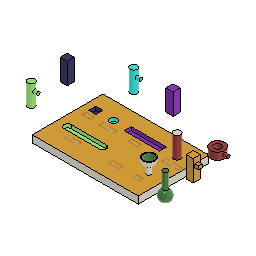
assembly_joint_practical (Autodesk Fusion 360 design; units mm, degrees)
part number: Joing-plate
part number: Rigid part
part number: Revolute part
part number: Slider part
part number: Cylindrical
part number: Pin-Slot part
part number: Planar part
part number: Ball part
Autodesk Fusion 360 part; units mm, degrees
sketch "スケッチ1" plane through (0, 0, 0) normal (0, 1, 0) x (1, 0, 0) in component "Joint-plate"
  line L0 (75, -50) -> (-75, -50)
  line L1 (-75, -50) -> (-75, 50)
  line L2 (-75, 50) -> (75, 50)
  line L3 (75, 50) -> (75, -50)
  line L4 (75, -50) -> (-75, 50) construction
  line L5 (-75, -50) -> (75, 50) construction
  dimension "d1" = 100
  dimension "d2" = 150
  constraint perpendicular L0 L1
  constraint parallel L0 L2
  constraint parallel L1 L3
  constraint horizontal L0
  constraint coincident L4 origin
  constraint coincident L5 origin
  measures "d1" distance of L0.end L1.end
  measures "d2" distance of L1.end L2.end
extrude "押し出し1" add sketch "スケッチ1" along normal blind 10 makes body 1 in component "Joint-plate"
sketch "スケッチ2" plane through (0, 10, 0) normal (0, 1, 0) x (-1, 0, 0) in component "Joint-plate"
  line L0 (-75, -50) -> (75, -50)
  line L1 (75, -50) -> (75, 50)
  line L2 (75, 50) -> (-75, 50)
  line L3 (-75, 50) -> (-75, -50)
  line L4 (65, -30) -> (55, -30)
  line L5 (55, -30) -> (55, -20)
  line L6 (55, -20) -> (65, -20)
  line L7 (65, -20) -> (65, -30)
  dimension "d5" = 10
  dimension "d6" = 20
  dimension "d7" = 10
  dimension "d8" = 10
  constraint horizontal L4
  constraint vertical L5
  constraint horizontal L6
  constraint vertical L7
  measures "d5" distance of L1 L7
  measures "d6" distance of L0 L4
  measures "d7" distance of L4.start L6.end
  measures "d8" distance of L5.end L6.end
extrude "押し出し2" cut sketch "スケッチ2" against normal blind 5 contours L4 L5 L6 L7 bodies 1 in component "Joint-plate"
sketch "スケッチ3" plane through (0, 10, 0) normal (0, 1, 0) x (-1, 0, 0) in component "Joint-plate"
  line L0 (55, -30) -> (55, -20)
  line L1 (55, -20) -> (65, -20)
  line L2 (65, -20) -> (65, -30)
  line L3 (65, -30) -> (55, -30)
  line L4 (-75, -50) -> (75, -50)
  line L5 (75, -50) -> (75, 50)
  line L6 (75, 50) -> (-75, 50)
  line L7 (-75, 50) -> (-75, -50)
  circle A0 centre (35, -25) radius 5
  dimension "d11" = 25
  dimension "d12" = 10
  dimension "d13" = 40
  measures "d11" distance of L4 A0.centre
  measures "d12" diameter of A0
  measures "d13" distance of L5 A0.centre
extrude "押し出し3" cut sketch "スケッチ3" against normal blind 5 contours A0 bodies 1 in component "Joint-plate"
sketch "スケッチ4" plane through (0, 10, 0) normal (0, 1, 0) x (-1, 0, 0) in component "Joint-plate"
  circle A0 centre (35, -25) radius 5
  line L0 (55, -30) -> (55, -20)
  line L1 (55, -20) -> (65, -20)
  line L2 (65, -20) -> (65, -30)
  line L3 (65, -30) -> (55, -30)
  line L4 (-75, -50) -> (75, -50)
  line L5 (75, -50) -> (75, 50)
  line L6 (75, 50) -> (-75, 50)
  line L7 (-75, 50) -> (-75, -50)
  line L8 (15, -30) -> (-35, -30)
  line L9 (-35, -30) -> (-35, -20)
  line L10 (-35, -20) -> (15, -20)
  line L11 (15, -20) -> (15, -30)
  dimension "d16" = 10
  dimension "d17" = 20
  dimension "d18" = 60
  dimension "d19" = 50
  constraint horizontal L8
  constraint vertical L9
  constraint horizontal L10
  constraint vertical L11
  measures "d16" distance of L8.start L10.end
  measures "d17" distance of L4 L8
  measures "d18" distance of L5 L11
  measures "d19" distance of L8.start L8.end
extrude "押し出し4" cut sketch "スケッチ4" against normal blind 5 contours L8 L9 L10 L11 bodies 1 in component "Joint-plate"
sketch "スケッチ5" plane through (0, 10, 0) normal (0, 1, 0) x (-1, 0, 0) in component "Joint-plate"
  line L0 (-35, -30) -> (-35, -20)
  line L1 (-35, -20) -> (15, -20)
  line L2 (15, -20) -> (15, -30)
  line L3 (15, -30) -> (-35, -30)
  circle A0 centre (35, -25) radius 5
  line L4 (55, -30) -> (55, -20)
  line L5 (55, -20) -> (65, -20)
  line L6 (65, -20) -> (65, -30)
  line L7 (65, -30) -> (55, -30)
  line L8 (-75, -50) -> (75, -50)
  line L9 (75, -50) -> (75, 50)
  line L10 (75, 50) -> (-75, 50)
  line L11 (-75, 50) -> (-75, -50)
  circle A1 centre (-55, -25) radius 5
  dimension "d22" = 20
  dimension "d23" = 10
  dimension "d24" = 25
  measures "d22" distance of L11 A1.centre
  measures "d23" diameter of A1
  measures "d24" distance of L8 A1.centre
extrude "押し出し5" add sketch "スケッチ5" along normal blind 30 contours A1 bodies 1 in component "Joint-plate"
sketch "スケッチ6" plane through (0, 10, 0) normal (0, 1, 0) x (-1, 0, 0) in component "Joint-plate"
  circle A0 centre (-55, -25) radius 5
  line L0 (-35, -30) -> (-35, -20)
  line L1 (-35, -20) -> (15, -20)
  line L2 (15, -20) -> (15, -30)
  line L3 (15, -30) -> (-35, -30)
  circle A1 centre (35, -25) radius 5
  line L4 (55, -30) -> (55, -20)
  line L5 (55, -20) -> (65, -20)
  line L6 (65, -20) -> (65, -30)
  line L7 (65, -30) -> (55, -30)
  line L8 (-75, -50) -> (75, -50)
  line L9 (75, -50) -> (75, 50)
  line L10 (75, 50) -> (-75, 50)
  line L11 (-75, 50) -> (-75, -50)
  line L12 (60, 20) -> (10, 20)
  arc A2 (10, 20) -> (10, 10) centre (10, 15) ccw
  line L13 (10, 10) -> (60, 10)
  arc A3 (60, 10) -> (60, 20) centre (60, 15) ccw
  line L14 (60, 15) -> (10, 15) construction
  dimension "d27" = 35
  dimension "d28" = 15
  dimension "d29" = 50
  dimension "d30" = 5
  constraint tangent L12 A2
  constraint tangent A2 L13
  constraint parallel L12 L13
  constraint tangent L13 A3
  constraint tangent L12 A3
  constraint perpendicular L9 L14
  measures "d27" distance of L10 L14
  measures "d28" distance of L9 A3.centre
  measures "d29" distance of A3.centre A2.centre
  measures "d30" radius of A3
extrude "押し出し6" cut sketch "スケッチ6" against normal blind 5 contours L12 A2 L13 A3 bodies 1 in component "Joint-plate"
ref_plane "作業平面1" through (-35, 7.5, 15) normal (0, 0, 1) x (-1, 0, 0) in component "Joint-plate"
sketch "スケッチ8" plane through (-35, 7.5, 15) normal (0, 0, 1) x (1, 0, 0) in component "Joint-plate"
  line L0 (90, 2.5) -> (87, 2.5)
  line L1 (87, 2.5) -> (87, 20.5)
  line L2 (87, 20.5) -> (90, 20.5)
  line L3 (90, 20.5) -> (90, 2.5)
  line L4 (85, 2.5) -> (95, 2.5)
  circle A0 centre (90, 20.5) radius 9
  line L5 (81.225, 22.5) -> (98.775, 22.5)
  circle A1 centre (90, 20.5) radius 8
  dimension "d33" = 1
  dimension "d34" = 18
  dimension "d35" = 18
  dimension "d36" = 3
  dimension "d37" = 2
  constraint horizontal L0
  constraint vertical L1
  constraint horizontal L2
  constraint vertical L3
  constraint midpoint L0.start L4
  constraint coincident L2.end L3.start
  constraint coincident A0 L5.start
  constraint coincident A0 L5.end
  constraint horizontal L5
  measures "d34" diameter of A0
  measures "d35" distance of L0.end L1.end
  measures "d36" distance of L1 L3
  measures "d37" distance of L5 L2.end
revolve "回転1" add sketch "スケッチ8" angle 360 about axis through (55, 28, 15) along (0, -1, 0) contours L0 L1 L3 L4 A0 | L1 L3 A0 A1 | L1 A0 L5 A1 bodies 1 in component "Joint-plate"
sketch "スケッチ9" plane through (0, 10, 0) normal (0, 1, 0) x (-1, 0, 0) in component "Joint-plate"
  line L0 (64.454, -10.2562) -> (53.8144, -10.2562) construction
  line L1 (53.8144, -10.2562) -> (53.8144, -15.2562) construction
  line L2 (53.8144, -15.2562) -> (64.454, -15.2562) construction
  line L3 (64.454, -15.2562) -> (64.454, -10.2562) construction
  line L4 (39.1349, -9.332) -> (20.0016, -9.332) construction
  line L5 (20.0016, -9.332) -> (20.0016, -14.332) construction
  line L6 (20.0016, -14.332) -> (39.1349, -14.332) construction
  line L7 (39.1349, -14.332) -> (39.1349, -9.332) construction
  line L8 (-1.2632, -10.1585) -> (-13.8902, -10.1585) construction
  line L9 (-13.8902, -10.1585) -> (-13.8902, -15.1585) construction
  line L10 (-13.8902, -15.1585) -> (-1.2632, -15.1585) construction
  line L11 (-1.2632, -15.1585) -> (-1.2632, -10.1585) construction
  line L12 (-48.8921, -10.1092) -> (-71.353, -10.1092) construction
  line L13 (-71.353, -10.1092) -> (-71.353, -15.1092) construction
  line L14 (-71.353, -15.1092) -> (-48.8921, -15.1092) construction
  line L15 (-48.8921, -15.1092) -> (-48.8921, -10.1092) construction
  line L16 (47.929, 30.2071) -> (30.844, 30.2071) construction
  line L17 (30.844, 30.2071) -> (30.844, 25.2071) construction
  line L18 (30.844, 25.2071) -> (47.929, 25.2071) construction
  line L19 (47.929, 25.2071) -> (47.929, 30.2071) construction
  line L20 (-48.7279, 30.2071) -> (-56.3475, 30.2071) construction
  line L21 (-56.3475, 30.2071) -> (-56.3475, 25.2071) construction
  line L22 (-56.3475, 25.2071) -> (-48.7279, 25.2071) construction
  line L23 (-48.7279, 25.2071) -> (-48.7279, 30.2071) construction
  line L24 (-13.7279, 30) -> (-27.8636, 30) construction
  line L25 (-27.8636, 30) -> (-27.8636, 25) construction
  line L26 (-27.8636, 25) -> (-13.7279, 25) construction
  line L27 (-13.7279, 25) -> (-13.7279, 30) construction
  constraint perpendicular L0 L1
  constraint parallel L1 L3
  constraint perpendicular L4 L5
  constraint parallel L4 L6
  constraint parallel L5 L7
  constraint perpendicular L8 L9
  constraint parallel L8 L10
  constraint parallel L9 L11
  constraint perpendicular L12 L13
  constraint parallel L12 L14
  constraint parallel L13 L15
  constraint perpendicular L16 L17
  constraint parallel L16 L18
  constraint parallel L17 L19
  constraint perpendicular L20 L21
  constraint parallel L20 L22
  constraint parallel L21 L23
  constraint perpendicular L24 L25
  constraint parallel L24 L26
  constraint parallel L25 L27
sketch "スケッチ1 (2)" plane through (0, 0, 0) normal (0, 1, 0) x (1, 0, 0) in component "Rigid part"
  line L0 (5, -5) -> (-5, -5)
  line L1 (-5, -5) -> (-5, 5)
  line L2 (-5, 5) -> (5, 5)
  line L3 (5, 5) -> (5, -5)
  line L4 (5, -5) -> (-5, 5) construction
  line L5 (-5, -5) -> (5, 5) construction
  dimension "d39" = 10
  dimension "d40" = 10
  constraint perpendicular L0 L1
  constraint parallel L0 L2
  constraint parallel L1 L3
  constraint horizontal L0
  constraint coincident L4 origin
  constraint coincident L5 origin
  measures "d39" distance of L1.end L2.end
  measures "d40" distance of L0.end L1.end
extrude "押し出し1'" add sketch "スケッチ1 (2)" along normal blind 30 separate body makes body 2 in component "Rigid part"
sketch "スケッチ1 (3)" plane through (0, 0, 0) normal (0, 1, 0) x (1, 0, 0) in component "Revolute part"
  circle A0 centre (0, 0) radius 5
  dimension "d43" = 10
  constraint coincident A0.centre origin
  measures "d43" diameter of A0
extrude "押し出し1''" add sketch "スケッチ1 (3)" along normal blind 30 separate body makes body 3 in component "Revolute part"
sketch "スケッチ2 (2)" plane through (0, 0, 0) normal (1, 0, 0) x (0, 0, -1) in component "Revolute part"
  line L0 (0, 30) -> (0, 0) construction
  circle A0 centre (0, 20) radius 2.5
  point P0 (0, 30)
  dimension "d46" = 5
  dimension "d47" = 20
  constraint coincident P0 L0.start
  constraint coincident L0.end origin
  constraint coincident L0 A0.centre
  measures "d46" diameter of A0
  measures "d47" distance of L0.end A0.centre
extrude "押し出し2'" add sketch "スケッチ2 (2)" along normal blind 10 bodies 3 in component "Revolute part"
sketch "スケッチ1 (4)" plane through (0, 0, 0) normal (0, 1, 0) x (1, 0, 0) in component "Slider part"
  line L0 (5, -5) -> (-5, -5)
  line L1 (-5, -5) -> (-5, 5)
  line L2 (-5, 5) -> (5, 5)
  line L3 (5, 5) -> (5, -5)
  line L4 (5, -5) -> (-5, 5) construction
  line L5 (-5, -5) -> (5, 5) construction
  dimension "d50" = 10
  dimension "d51" = 10
  constraint perpendicular L0 L1
  constraint parallel L0 L2
  constraint parallel L1 L3
  constraint horizontal L0
  constraint coincident L4 origin
  constraint coincident L5 origin
  measures "d50" distance of L1.end L2.end
  measures "d51" distance of L0.end L1.end
extrude "押し出し1'''" add sketch "スケッチ1 (4)" along normal blind 30 separate body makes body 4 in component "Slider part"
sketch "スケッチ1 (5)" plane through (0, 0, 0) normal (0, 1, 0) x (1, 0, 0) in component "Cylinderical"
  circle A0 centre (0, 0) radius 10
  circle A1 centre (0, 0) radius 5
  dimension "d54" = 10
  dimension "d55" = 5
  constraint coincident A0.centre A1.centre
  measures "d54" diameter of A1
  measures "d55" distance of A0 A1
extrude "押し出し1''''" add sketch "スケッチ1 (5)" along normal blind 10 separate body makes body 5 in component "Cylinderical"
sketch "スケッチ2 (3)" plane through (0, 0, 0) normal (1, 0, 0) x (0, 0, -1) in component "Cylinderical"
  line L0 (10, 10) -> (-10, 10)
  line L1 (0, 10) -> (0, 0) construction
  circle A0 centre (0, 5) radius 2.5
  dimension "d58" = 5
  constraint midpoint L0 L1.start
  constraint coincident L1.end origin
  constraint midpoint L1 A0.centre
  measures "d58" diameter of A0
extrude "押し出し2''" add sketch "スケッチ2 (3)" along normal blind 15 bodies 5 in component "Cylinderical"
delete_face "面を削除1" 1 faces at (1.6667, 7.5, 0) on bodies 5 in component "Cylinderical"
sketch "スケッチ1 (6)" plane through (0, 0, 0) normal (0, 1, 0) x (1, 0, 0) in component "Pin-Slot part"
  circle A0 centre (0, 0) radius 5
  dimension "d61" = 10
  constraint coincident A0.centre origin
  measures "d61" diameter of A0
extrude "押し出し1'''''" add sketch "スケッチ1 (6)" along normal blind 30 separate body makes body 6 in component "Pin-Slot part"
sketch "スケッチ2 (4)" plane through (0, 0, 0) normal (1, 0, 0) x (0, 0, -1) in component "Pin-Slot part"
  line L0 (0, 30) -> (0, 0) construction
  circle A0 centre (0, 20) radius 2.5
  point P0 (0, 30)
  dimension "d64" = 5
  dimension "d65" = 20
  constraint coincident P0 L0.start
  constraint coincident L0.end origin
  constraint coincident L0 A0.centre
  measures "d64" diameter of A0
  measures "d65" distance of L0.end A0.centre
extrude "押し出し2'''" add sketch "スケッチ2 (4)" along normal blind 10 bodies 6 in component "Pin-Slot part"
sketch "スケッチ1 (7)" plane through (0, 0, 0) normal (0, 1, 0) x (1, 0, 0) in component "Planar part"
  line L0 (5, -5) -> (-5, -5)
  line L1 (-5, -5) -> (-5, 5)
  line L2 (-5, 5) -> (5, 5)
  line L3 (5, 5) -> (5, -5)
  line L4 (5, -5) -> (-5, 5) construction
  line L5 (-5, -5) -> (5, 5) construction
  dimension "d68" = 10
  dimension "d69" = 10
  constraint perpendicular L0 L1
  constraint parallel L0 L2
  constraint parallel L1 L3
  constraint horizontal L0
  constraint coincident L4 origin
  constraint coincident L5 origin
  measures "d68" distance of L0.end L1.end
  measures "d69" distance of L1.end L2.end
extrude "押し出し1''''''" add sketch "スケッチ1 (7)" along normal blind 30 separate body makes body 7 in component "Planar part"
sketch "スケッチ2 (5)" plane through (5, 0, 0) normal (1, 0, 0) x (0, 0, -1) in component "Planar part"
  line L0 (-5, 0) -> (5, 0)
  line L1 (5, 0) -> (5, 30)
  line L2 (5, 30) -> (-5, 30)
  line L3 (-5, 30) -> (-5, 0)
  line L4 (0, 30) -> (0, 0) construction
  line L5 (2.5, 17.5) -> (-2.5, 17.5)
  line L6 (-2.5, 17.5) -> (-2.5, 22.5)
  line L7 (-2.5, 22.5) -> (2.5, 22.5)
  line L8 (2.5, 22.5) -> (2.5, 17.5)
  line L9 (2.5, 17.5) -> (-2.5, 22.5) construction
  line L10 (-2.5, 17.5) -> (2.5, 22.5) construction
  point P0 (0, 20)
  dimension "d72" = 5
  dimension "d73" = 5
  dimension "d74" = 20
  constraint midpoint L2 L4.start
  constraint coincident L4.end origin
  constraint perpendicular L5 L6
  constraint parallel L5 L7
  constraint parallel L6 L8
  constraint horizontal L5
  constraint coincident L9 P0
  constraint coincident L10 P0
  constraint coincident L4 P0
  measures "d72" distance of L6.end L7.end
  measures "d73" distance of L5.end L6.end
  measures "d74" distance of L0 P0
extrude "押し出し2''''" add sketch "スケッチ2 (5)" along normal blind 5 contours L5 L6 L7 L8 bodies 7 in component "Planar part"
sphere "球プリミティブ1" add diameter 17 placed x (1, 0, 0) y (0, 0, -1) z (0, 1, 0) at (0, 0, 0) separate body makes body 8 in component "Ball part"
cylinder "円柱プリミティブ1" add diameter 7 height 30 placed x (1, 0, 0) y (0, 0, -1) z (0, 1, 0) at (0, 0, 0) bodies 8 in component "Ball part"
component "Joint-plate" placed x (1, 0, 0) y (0, 0, 1) z (0, -1, 0) at (0, 0, 0)
component "Rigid part" placed x (1, 0, 0) y (0, 0, 1) z (0, -1, 0) at (-102.7267, 27.1916, 22.5212)
component "Revolute part" placed x (1, 0, 0) y (0, 0, 1) z (0, -1, 0) at (-37.7234, 56.3901, 28.2574)
component "Slider part" placed x (1, 0, 0) y (0, 0, 1) z (0, -1, 0) at (15.5955, 58.5659, 28.4948)
component "Cylinderical" placed x (1, 0, 0) y (0, 0, -1) z (0, 1, 0) at (100.0865, 37.2295, 39.7051)
component "Pin-Slot part" placed x (1, 0, 0) y (0, 0, 1) z (0, -1, 0) at (-98.7244, -27.7459, 22.9507)
component "Planar part" placed x (1, 0, 0) y (0, 0, 1) z (0, -1, 0) at (102.4888, 0.229, 19.4212)
component "Ball part" placed x (1, 0, 0) y (0, 0, 1) z (0, -1, 0) at (103.0529, -39.864, 20.1832)
